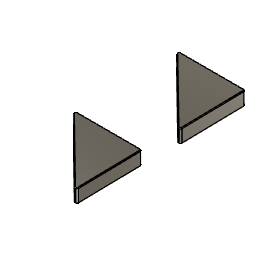
Frame Holder (Autodesk Fusion 360 design; units mm, degrees)
Autodesk Fusion 360 part; units mm, degrees
sketch "Sketch1" plane through (0, 0, 0) normal (0, 0, 1) x (1, 0, 0)
  line L0 (0, 0) -> (50, 0)
  line L1 (50, 0) -> (50.9223, -49.9915)
  line L2 (50.9223, -49.9915) -> (0, 0)
  line L3 (2.4461, -1) -> (49.0183, -1)
  line L4 (49.0183, -1) -> (49.8773, -47.5643)
  line L5 (49.8773, -47.5643) -> (2.4461, -1)
  dimension "d1" = 50
  dimension "d2" = 50
  dimension "d3" = 1
  constraint coincident L0.start L2.end
  constraint horizontal L0
  measures "d1" distance of L0.start L0.end
  measures "d2" distance of L0.end L1.end
extrude "Extrude1" add sketch "Sketch1" along normal blind 10 contours L0 L1 L2 | L3 L4 L5 makes body 1
shell "Shell1" thickness 1 removed faces 1 at (33.9482, -33.3277, 3.3333) on bodies 1
fillet "Fillet1" radius 1.25 1 edges at (0, 0, 5) on bodies 1
fillet "Fillet2" radius 1.25 1 edges at (50.9223, -49.9915, 5) on bodies 1
fillet "Fillet3" radius 1.25 1 edges at (50, 0, 5) on bodies 1
fillet "Fillet4" radius 0.5 12 edges at (49.6485, -0.358, 10) (25.9152, 0, 10) (1.9005, -0.777, 10) (25.4611, -24.9957, 10) (50.1104, -48.1056, 10) (50.4442, -24.0807, 10) (25.9152, 0, 0) (1.9005, -0.777, 0) (25.4611, -24.9957, 0) (50.1104, -48.1056, 0) (50.4442, -24.0807, 0) (49.6485, -0.358, 0) on bodies 1
copy_body "CopyPasteBodies1" bodies 1 makes body 2
move_body "Move1" bodies 2 to x (1, 0, 0) y (0, 1, 0) z (0, 0, 1) at (0, -75, 0)
extrude "Extrude2" cut 1 faces at (18.296, 0, 3.5) along direction (0, -1, 0) blind 1 on bodies 1 bodies 1
extrude "Extrude3" cut 1 faces at (2.2411, -1, 6.3333) along direction (0, 1, 0) blind 3 on bodies 1 bodies 1
extrude "Extrude4" add 1 faces at (18.296, -0.3333, 0.5) along direction (0, 0, 1) blind 0.5 on bodies 1 bodies 1
extrude "Extrude5" add 1 faces at (18.296, -0.3333, 9.5) along direction (0, 0, -1) blind 0.5 on bodies 1 bodies 1
